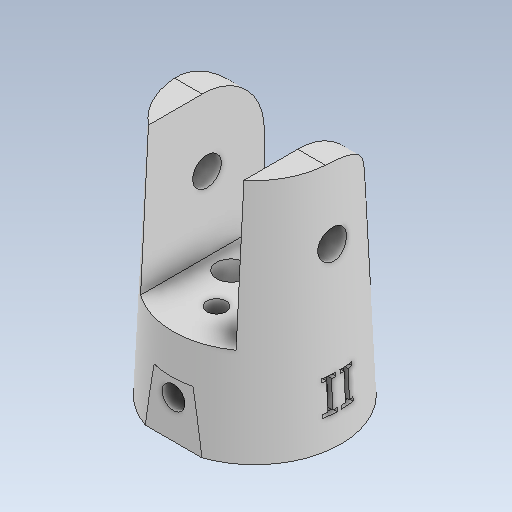
# Autodesk Inventor part: Bauteil2
Saved by Autodesk Inventor 2021 (Build 250183000, 183)
## iProperties
Created: 2021-04-30
Part Number: Bauteil2
Material: Generisch
Document SubType Name: Modeling
Designer: Maxim
Density: 1 g/cm^3
Appearance: Vorgabe
Author: Maxim
Autodesk Inventor part; units mm, degrees
ref_plane "XZ Plane" through (0, 0, 0) normal (0, 1, 0) x (-1, 0, 0)
sketch "Skizze1" plane through (0, 0, 0) normal (0, 1, 0) x (-1, 0, 0)
  circle A0 centre (0, 0) radius 9
  dimension "d6" = 18
  constraints: 1 centre point
  measures "d6" diameter of A0
extrude "Extrusion1" add sketch "Skizze1" along normal blind 25
draft "Flächenverjüngung1" angle -2.5 pull direction (0, -1, 0) faces at (-8.8835, 8.3333, -1.4437) fixed edges at (9, 0, 0)
sketch "Skizze2" plane through (0, 25, 0) normal (0, 1, 0) x (1, 0, 0)
  line L0 (-5, 13.1758) -> (5, 13.1758)
  line L1 (5, 13.1758) -> (5, -14.5696)
  line L2 (5, -14.5696) -> (-5, -14.5696)
  line L3 (-5, -14.5696) -> (-5, 13.1758)
  circle A0 centre (0, 0) radius 9 projected
  point P0 (5, -7.4833)
  point P1 (-5, -7.4833)
  point P2 (-5, 7.4833)
  point P3 (5, 7.4833)
  dimension "d14" = 10
  dimension "d15" = 5
  constraints: 8 end point, 2 parallel, 1 horizontal, 1 perpendicular
  measures "d14" distance of L0.start L0.end
  measures "d15" distance from line of A0.centre L1
extrude "Extrusion2" cut sketch "Skizze2" against normal blind 15 contours L0 L1 A0 L3 | A0 L1 L3 | A0 L1 L2 L3
sketch "Skizze3" plane through (0, 0, 0) normal (1, 0, 0) x (0, 1, 0)
  circle A0 centre (17.75, 0) radius 1.5
  line L0 (0, 8.657) -> (0, -8.657) projected
  line L1 (25, -6.1273) -> (25, 6.1273) projected
  line L2 (-4.8, 0) -> (28.8, 0) projected
  point P0 (0, 0)
  dimension "d16" = 3
  dimension "d46" = 7.25
  dimension "d66" = 0
  constraints: 1 centre point
  measures "d16" diameter of A0
  measures "d46" distance from line of L1 A0.centre
  measures "d66" distance from line of L2 A0.centre
extrude "Extrusion3" cut sketch "Skizze3" along normal mid plane 30
sketch "Skizze5" plane through (0, 0, 0) normal (1, 0, 0) x (0, 1, 0)
  line L0 (36.5276, -18.963) -> (10, -18.963)
  line L1 (10, -18.963) -> (10, -6)
  line L2 (10, -6.9521) -> (10, 6.9521) projected
  line L3 (10, -6) -> (25, -6)
  line L4 (25, -6.1273) -> (25, 6.1273) projected
  line L5 (25, -6) -> (25, 10.0811)
  line L6 (25, 10.0811) -> (36.5276, 10.0811)
  line L7 (36.5276, 10.0811) -> (36.5276, -18.963)
  line L8 (-7.1055, 0) -> (42.6331, 0) projected
  point P0 (0, 0)
  point P1 (25, -4.5049)
  dimension "d52" = 6
  constraints: 12 end point, 3 perpendicular, 2 point on line, 1 horizontal, 1 vertical
  measures "d52" distance between parallel lines of L8 L3
extrude "Extrusion9" add sketch "Skizze5" along normal mid plane 30 separate body contours L0 L1 L3 L4 L8 L7 | L8 L4 L5 L6 L7
fillet "Rundung3" radius 6.5 1 edges at (0, 25, -6)
combine bodies "Kombinieren2" operation type subtract main body 1 bodies to subtract 2
sketch "Skizze7" plane through (0, 0, 0) normal (1, 0, 0) x (0, 1, 0)
  line L0 (-3.7576, 12.594) -> (6, 12.594)
  line L1 (6, 12.594) -> (6, 8.5)
  line L2 (6, 8.5) -> (-3.7576, 8.5)
  line L3 (-3.7576, 8.5) -> (-3.7576, 12.594)
  line L4 (0, -9) -> (0, 9) projected
  line L5 (-5.7092, 0) -> (7.9515, 0) projected
  point P0 (0, 0)
  dimension "d47" = 6
  dimension "d48" = 8.5
  constraints: 8 end point, 2 parallel, 1 horizontal, 1 perpendicular
  measures "d47" distance between parallel lines of L4 L1
  measures "d48" distance between parallel lines of L5 L2
extrude "Extrusion10" add sketch "Skizze7" along normal mid plane 40 separate body
combine bodies "Kombinieren4" operation type subtract main body 1 bodies to subtract 3
sketch "Skizze8" plane through (0, 0, 0) normal (0, 1, 0) x (-1, 0, 0)
  circle A0 centre (0, 4) radius 1
  line L0 (0, -1) -> (0, 6) projected
  line L1 (-1.4, 0) -> (1.4, 0) projected
  point P0 (0, 0)
  point P1 (0, 5)
  point P2 (0, 3)
  dimension "d53" = 0
  dimension "d55" = 2
  dimension "d76" = 4
  constraints: 1 centre point
  measures "d53" distance from line of L0 A0.centre
  measures "d55" diameter of A0
  measures "d76" distance from line of L1 A0.centre
extrude "Extrusion11" add sketch "Skizze8" along normal blind 22.25 separate body
combine bodies "Kombinieren5" operation type subtract main body 1 bodies to subtract 4
ref_plane "Arbeitsebene1" through (0, 0, 5.5) normal (0, 0, 1) x (1, 0, 0)
sketch "Skizze9" plane through (0, 0, 5.5) normal (0, 0, 1) x (1, 0, 0)
  circle A0 centre (0, 4) radius 1.2
  line L0 (-1.68, 0) -> (1.68, 0) projected
  point P0 (0, 0)
  dimension "d60" = 2.4
  dimension "d61" = 4
  constraints: 1 centre point
  measures "d60" diameter of A0
  measures "d61" distance from line of L0 A0.centre
extrude "Extrusion12" add sketch "Skizze9" along normal blind 22.25 separate body
combine bodies "Kombinieren6" operation type subtract main body 1 bodies to subtract 5
sketch "Skizze11" plane through (0, 0, 0) normal (0, 1, 0) x (-1, 0, 0)
  circle A0 centre (-2.5, 0) radius 1.5
  circle A1 centre (2.5, 0) radius 1.5
  line L0 (0, -2.1) -> (0, 2.1) projected
  line L1 (-5.7, 0) -> (6.2, 0) projected
  point P0 (4, 0)
  point P1 (1, 0)
  point P2 (-4, 0)
  point P3 (-1, 0)
  dimension "d70" = 3
  dimension "d71" = 3
  dimension "d72" = 2.5
  dimension "d73" = 0
  dimension "d74" = 2.5
  dimension "d75" = 0
  constraints: 2 centre point
  measures "d70" diameter of A0
  measures "d71" diameter of A1
  measures "d72" distance from line of L0 A1.centre
  measures "d73" distance from line of L1 A1.centre
  measures "d74" distance from line of L0 A0.centre
  measures "d75" distance from line of L1 A0.centre
extrude "Extrusion13" add sketch "Skizze11" along normal blind 15 separate body
combine bodies "Kombinieren7" operation type subtract main body 1 bodies to subtract 6
ref_plane "Arbeitsebene2" through (9, 0, 0) normal (1, 0, 0) x (0, 1, 0)
sketch "Skizze12" plane through (9, 0, 0) normal (1, 0, 0) x (0, 1, 0)
  line L0 (6.5, 1.8) -> (6.5, -1.7) construction
  line L1 (6.5, -1.7) -> (3, -1.7) construction
  line L2 (3, -1.7) -> (3, 1.8) construction
  line L3 (3, 1.8) -> (6.5, 1.8) construction
  line L4 (-1.7, 0) -> (10.2, 0) projected
  line L5 (0, 2.5) -> (0, -2.4) projected
  line L6 (3, 0.2259) -> (3, 1.5816)
  line L7 (3, 1.5816) -> (3.3574, 1.5816)
  line L8 (3.3574, 1.5816) -> (3.3574, 1.1363)
  line L9 (3.3574, 1.1363) -> (6.1426, 1.1363)
  line L10 (6.1426, 1.1363) -> (6.1426, 1.5816)
  line L11 (6.1426, 1.5816) -> (6.5, 1.5816)
  line L12 (6.5, 1.5816) -> (6.5, 0.2259)
  line L13 (6.5, 0.2259) -> (6.1426, 0.2259)
  line L14 (6.1426, 0.2259) -> (6.1426, 0.6712)
  line L15 (6.1426, 0.6712) -> (3.3574, 0.6712)
  line L16 (3.3574, 0.6712) -> (3.3574, 0.2259)
  line L17 (3.3574, 0.2259) -> (3, 0.2259)
  line L18 (3, -1.5695) -> (3, -0.2138)
  line L19 (3, -0.2138) -> (3.3574, -0.2138)
  line L20 (3.3574, -0.2138) -> (3.3574, -0.6591)
  line L21 (3.3574, -0.6591) -> (6.1426, -0.6591)
  line L22 (6.1426, -0.6591) -> (6.1426, -0.2138)
  line L23 (6.1426, -0.2138) -> (6.5, -0.2138)
  line L24 (6.5, -0.2138) -> (6.5, -1.5695)
  line L25 (6.5, -1.5695) -> (6.1426, -1.5695)
  line L26 (6.1426, -1.5695) -> (6.1426, -1.1242)
  line L27 (6.1426, -1.1242) -> (3.3574, -1.1242)
  line L28 (3.3574, -1.1242) -> (3.3574, -1.5695)
  line L29 (3.3574, -1.5695) -> (3, -1.5695)
  point P0 (0, 0)
  dimension "d78" = 3.5
  dimension "d79" = 3.5
  dimension "d80" = 1.8
  dimension "d83" = 3
  constraints: 2 other
  measures "d78" distance of L2.end L0.start
  measures "d79" distance of L0.start L0.end
  measures "d80" distance between parallel lines of L4 L3
  measures "d83" distance between parallel lines of L5 L2
emboss "Prägen1" sketch "Skizze12" operation cut depth 0.5 direction (-1, 0, 0)
